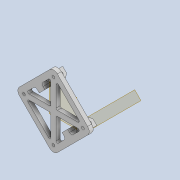
# Autodesk Inventor part: base_stand_1
Saved by Autodesk Inventor 2020 (Build 240168000, 168)
## iProperties
Created: 2021-09-25
Part Number: base_stand_1
Material: Generic
Document SubType Name: Modeling
Designer: Shuang Peng
Density: 1 g/cm^3
Appearance: Default
Author: Shuang Peng
Autodesk Inventor part; units mm, degrees
ref_plane "YZ Plane" through (0, 0, 0) normal (1, 0, 0) x (0, 1, 0)
ref_plane "XZ Plane" through (0, 0, 0) normal (0, 1, 0) x (-1, 0, 0)
ref_plane "XY Plane" through (0, 0, 0) normal (0, 0, 1) x (1, 0, 0)
ref_plane "Work Plane1" through (0, 0, 10) normal (0, 0, 1) x (1, 0, 0)
sketch "Sketch1" plane through (0, 0, 10) normal (0, 0, 1) x (1, 0, 0)
  circle A0 centre (0, 0) radius 1.5 projected
  line L0 (-11.1464, -3.182) -> (-3.182, -11.1464) projected
  line L1 (28.2843, 0) -> (0, -28.2843)
  line L2 (0, -28.2843) -> (-28.2843, 0)
  line L3 (-28.2843, 0) -> (0, 28.2843)
  line L4 (0, 28.2843) -> (28.2843, 0)
  line L5 (28.2843, 0) -> (-28.2843, 0) construction
  line L6 (0, -28.2843) -> (0, 28.2843) construction
  line L7 (22.6274, 0) -> (0, -22.6274)
  line L8 (0, -22.6274) -> (-22.6274, 0)
  line L9 (-22.6274, 0) -> (0, 22.6274)
  line L10 (0, 22.6274) -> (22.6274, 0)
  line L11 (22.6274, 0) -> (-22.6274, 0) construction
  line L12 (0, -22.6274) -> (0, 22.6274) construction
  point P0 (0, 0)
  dimension "d0" = 40
  dimension "d1" = 40
  dimension "d2" = 4
  dimension "d3" = 4
  constraints: 24 end point, 5 parallel, 4 midpoint, 2 perpendicular
  measures "d0" distance of L1.start L1.end
  measures "d1" distance of L1.end L2.end
  measures "d2" distance between parallel lines of L2 L8
  measures "d3" distance between parallel lines of L1 L7
extrude "Extrusion1" add sketch "Sketch1" along normal blind 3 contours L1 L2 L3 L4
ref_plane "Work Plane2" through (8.4853, -12.7279, -19) normal (0.7071068, 0.7071068, 0) x (-0.7071068, 0.7071068, 0)
sketch "Sketch2" plane through (8.4853, -12.7279, -19) normal (0.7071068, 0.7071068, 0) x (-0.7071068, 0.7071068, 0)
  circle A0 centre (30.0659, 17.5) radius 1 projected
  circle A1 centre (-0.0659, 17.5) radius 1 projected
  line L0 (33.0659, 14.5) -> (27.0659, 14.5)
  line L1 (27.0659, 14.5) -> (27.0659, 20.5)
  line L2 (27.0659, 20.5) -> (33.0659, 20.5)
  line L3 (33.0659, 20.5) -> (33.0659, 14.5)
  line L4 (33.0659, 14.5) -> (27.0659, 20.5) construction
  line L5 (27.0659, 14.5) -> (33.0659, 20.5) construction
  line L6 (-3.0659, 14.5) -> (2.9341, 14.5)
  line L7 (2.9341, 14.5) -> (2.9341, 20.5)
  line L8 (2.9341, 20.5) -> (-3.0659, 20.5)
  line L9 (-3.0659, 20.5) -> (-3.0659, 14.5)
  line L10 (-3.0659, 14.5) -> (2.9341, 20.5) construction
  line L11 (2.9341, 14.5) -> (-3.0659, 20.5) construction
  point P0 (15, 19)
  dimension "d6" = 6
  dimension "d7" = 6
  dimension "d8" = 6
  dimension "d9" = 6
  constraints: 24 end point, 4 midpoint, 4 parallel, 2 horizontal, 2 perpendicular
  measures "d6" distance of L0.start L0.end
  measures "d7" distance of L0.end L1.end
  measures "d8" distance of L6.start L6.end
  measures "d9" distance of L7.end L6.end
extrude "Extrusion2" add sketch "Sketch2" along normal blind 6
sketch "Sketch3" plane through (-10.6532, 6.4105, 1.5) normal (0, 0, 1) x (0.7071068, 0.7071068, 0)
  line L0 (0, 6) -> (0, 0) projected
  line L1 (0, 0) -> (6, 0) projected
  line L2 (6, 6) -> (6, 0) projected
  line L3 (0, 6) -> (6, 6) projected
  line L4 (0, -24.1317) -> (0, -30.1317) projected
  line L5 (0, -30.1317) -> (6, -30.1317) projected
  line L6 (6, -24.1317) -> (6, -30.1317) projected
  line L7 (0, -24.1317) -> (6, -24.1317) projected
  point P0 (3, -12.0659)
extrude "Extrusion3" add sketch "Sketch3" along normal up to surface (11.5 mm away)
sketch "Sketch4" plane through (0, 0, 13) normal (0, 0, 1) x (1, 0, 0)
  line L0 (-9.1924, 13.435) -> (0, 22.6274) projected
  line L1 (0, 22.6274) -> (22.6274, 0) projected
  line L2 (22.6274, 0) -> (13.435, -9.1924) projected
  line L3 (10.6532, -6.4105) -> (13.435, -9.1924) projected
  line L4 (6.4105, -10.6532) -> (10.6532, -6.4105) projected
  line L5 (9.1924, -13.435) -> (6.4105, -10.6532) projected
  line L6 (9.1924, -13.435) -> (0, -22.6274) projected
  line L7 (0, -22.6274) -> (-22.6274, 0) projected
  line L8 (-22.6274, 0) -> (-13.435, 9.1924) projected
  line L9 (-10.6532, 6.4105) -> (-13.435, 9.1924) projected
  line L10 (-6.4105, 10.6532) -> (-10.6532, 6.4105) projected
  line L11 (-9.1924, 13.435) -> (-6.4105, 10.6532) projected
  line L12 (0, -28.2843) -> (28.2843, 0) projected
  line L13 (28.2843, 0) -> (0, 28.2843) projected
  line L14 (0, 28.2843) -> (-28.2843, 0) projected
  line L15 (-28.2843, 0) -> (0, -28.2843) projected
  line L16 (0, -22.6274) -> (-22.6274, 0) projected
  line L17 (22.6274, 0) -> (13.435, -9.1924) projected
  line L18 (-22.6274, 0) -> (22.6274, 0) construction
  line L19 (-22.6274, -2) -> (22.6274, -2)
  line L20 (22.6274, 2) -> (-22.6274, 2)
  arc A0 (-22.6274, 2) -> (-22.6274, -2) centre (-22.6274, 0) ccw
  arc A1 (22.6274, -2) -> (22.6274, 2) centre (22.6274, 0) ccw
  line L21 (0, 22.6274) -> (22.6274, 0) projected
  line L22 (0, 22.6274) -> (0, -22.6274) construction
  line L23 (-2, 22.6274) -> (-2, -22.6274)
  line L24 (2, -22.6274) -> (2, 22.6274)
  arc A2 (2, 22.6274) -> (-2, 22.6274) centre (0, 22.6274) ccw
  arc A3 (-2, -22.6274) -> (2, -22.6274) centre (0, -22.6274) ccw
  point P0 (0, 0)
  point P1 (0, 0)
  point P2 (0, 0)
  point P3 (2, -2)
  point P4 (2, 2)
  point P5 (-2, 2)
  point P6 (-2, -2)
  dimension "d14" = 4
  dimension "d15" = 4
  constraints: 16 end point, 8 point on circle, 8 tangent, 4 centre point, 2 midpoint, 2 parallel, 1 horizontal, 1 vertical
  measures "d14" diameter of A1
  measures "d15" diameter of A3
extrude "Extrusion4" add sketch "Sketch4" against normal up to surface (3 mm away) contours L23 A2 L24 L1 L0 | L0 L1 L24 L20 L23 | L23 L19 L7 L8 L20 | L20 L24 L19 L23 | L20 L1 L2 L19 L24 | L8 L7 L19 A0 L20 | L19 L24 L6 L7 L23 | L20 A1 L19 L2 L1 | L7 L6 L24 A3 L23
fillet "Fillet1" radius 8 2 edges at (-12.7745, 12.7745, 10) (12.7745, -12.7745, 10)
fillet "Fillet2" radius 2 8 edges at (-10.6066, 14.8492, 10) (-9.1924, 13.435, 11.5) (13.435, -9.1924, 11.5) (14.8492, -10.6066, 10) (10.6066, -14.8492, 10) (9.1924, -13.435, 11.5) (-13.435, 9.1924, 11.5) (-14.8492, 10.6066, 10)
chamfer "Chamfer1" distance 2 angle 45 2 edges at (8.5319, -8.5319, -4.5) (-8.5319, 8.5319, -4.5)
fillet "Fillet3" radius 1 12 edges at (20.6274, -2, 11.5) (20.6274, 2, 11.5) (2, 2, 11.5) (2, 20.6274, 11.5) (-2, 20.6274, 11.5) (-20.6274, 2, 11.5) (-2, 2, 11.5) (2, -2, 11.5) (-2, -2, 11.5) (2, -20.6274, 11.5) (-2, -20.6274, 11.5) (-20.6274, -2, 11.5)
sketch "Sketch5" plane through (0, 0, 10) normal (0, 0, -1) x (-1, 0, 0)
  line L0 (14.8492, 7.7782) -> (17.6777, 10.6066) projected
  line L1 (18.9203, 3.7071) -> (14.8492, 7.7782) projected
  arc A0 (18.2132, 2) -> (18.9203, 3.7071) centre (18.2132, 3) ccw projected
  line L2 (18.2132, 2) -> (3, 2) projected
  arc A1 (2, 3) -> (3, 2) centre (3, 3) ccw projected
  line L3 (2, 3) -> (2, 18.2132) projected
  arc A2 (3.7071, 18.9203) -> (2, 18.2132) centre (3, 18.2132) ccw projected
  line L4 (7.7782, 14.8492) -> (3.7071, 18.9203) projected
  line L5 (10.6066, 17.6777) -> (7.7782, 14.8492) projected
  line L6 (0, 28.2843) -> (10.6066, 17.6777) projected
  line L7 (-28.2843, 0) -> (0, 28.2843) projected
  line L8 (-17.6777, -10.6066) -> (-28.2843, 0) projected
  line L9 (-14.8492, -7.7782) -> (-17.6777, -10.6066) projected
  line L10 (-18.9203, -3.7071) -> (-14.8492, -7.7782) projected
  arc A3 (-18.2132, -2) -> (-18.9203, -3.7071) centre (-18.2132, -3) ccw projected
  line L11 (-18.2132, -2) -> (-3, -2) projected
  arc A4 (-2, -3) -> (-3, -2) centre (-3, -3) ccw projected
  line L12 (-2, -3) -> (-2, -18.2132) projected
  arc A5 (-3.7071, -18.9203) -> (-2, -18.2132) centre (-3, -18.2132) ccw projected
  line L13 (-7.7782, -14.8492) -> (-3.7071, -18.9203) projected
  line L14 (-10.6066, -17.6777) -> (-7.7782, -14.8492) projected
  line L15 (0, -28.2843) -> (-10.6066, -17.6777) projected
  line L16 (28.2843, 0) -> (0, -28.2843) projected
  line L17 (17.6777, 10.6066) -> (28.2843, 0) projected
  arc A6 (2, -18.2132) -> (3.7071, -18.9203) centre (3, -18.2132) ccw projected
  line L18 (2, -18.2132) -> (2, -3) projected
  arc A7 (3, -2) -> (2, -3) centre (3, -3) ccw projected
  line L19 (3, -2) -> (18.2132, -2) projected
  arc A8 (18.9203, -3.7071) -> (18.2132, -2) centre (18.2132, -3) ccw projected
  line L20 (3.7071, -18.9203) -> (18.9203, -3.7071) projected
  line L21 (-2, 18.2132) -> (-2, 3) projected
  arc A9 (-3, 2) -> (-2, 3) centre (-3, 3) ccw projected
  line L22 (-3, 2) -> (-18.2132, 2) projected
  arc A10 (-18.9203, 3.7071) -> (-18.2132, 2) centre (-18.2132, 3) ccw projected
  line L23 (-3.7071, 18.9203) -> (-18.9203, 3.7071) projected
  arc A11 (-2, 18.2132) -> (-3.7071, 18.9203) centre (-3, 18.2132) ccw projected
  line L24 (0, 0) -> (22, 0)
  line L25 (-18.2132, -2) -> (-3, -2) projected
  circle A12 centre (22, 0) radius 1
  line L26 (0, 0) -> (-22, 0)
  line L27 (0, 0) -> (0, 22)
  line L28 (0, 0) -> (0, -22)
  circle A13 centre (0, -22) radius 1
  circle A14 centre (-22, 0) radius 1
  circle A15 centre (0, 22) radius 1
  dimension "d24" = 22
  dimension "d25" = 2
  dimension "d26" = 22
  dimension "d27" = 22
  dimension "d28" = 22
  dimension "d29" = 2
  dimension "d30" = 2
  dimension "d31" = 2
  constraints: 8 end point, 4 centre point, 4 coincident, 2 vertical, 1 horizontal, 1 parallel
  measures "d24" distance of L24.start L24.end
  measures "d25" diameter of A12
  measures "d26" distance of L24.start L26.end
  measures "d27" distance of L24.start L27.end
  measures "d28" distance of L24.start L28.end
  measures "d29" diameter of A13
  measures "d30" diameter of A14
  measures "d31" diameter of A15
extrude "Extrusion5" cut sketch "Sketch5" against normal blind 6 contours A12 | A13 | A14 | A15
fillet "Fillet4" radius 4 4 edges at (28.2843, 0, 11.5) (0, 28.2843, 11.5) (-28.2843, 0, 11.5) (0, -28.2843, 11.5)
body "Solid1"
